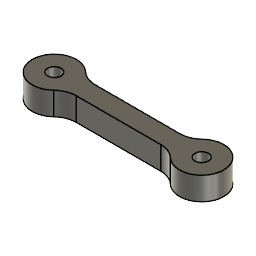
ConnectingBracketV0_v1 (Autodesk Fusion 360 design; units mm, degrees)
Autodesk Fusion 360 part; units mm, degrees
sketch "Sketch1" plane through (0, 0, 0) normal (0, 0, 1) x (1, 0, 0)
  line L0 (0, 0) -> (-19.119, 0) construction
  circle A0 centre (-19.119, 0) radius 0.875
  circle A1 centre (0, 0) radius 0.875
  line L1 (-9.5595, 0) -> (-9.5595, 1.25) construction
  line L2 (-9.5595, 0) -> (-9.5595, -1.25) construction
  line L3 (-19.119, 0) -> (-19.119, 0.875) construction
  line L4 (-19.119, 0.875) -> (-19.119, 2.875) construction
  circle A2 centre (-19.119, 0) radius 2.875
  line L5 (0, 0) -> (0, 0.875) construction
  line L6 (0, 0.875) -> (0, 2.875) construction
  circle A3 centre (0, 0) radius 2.875
  line L7 (-16.5237, 1.237) -> (-2.5953, 1.237)
  line L8 (-2.5953, 1.237) -> (-2.5953, -1.237) construction
  line L9 (-2.5953, -1.237) -> (-16.5237, -1.237)
  line L10 (-16.5237, -1.237) -> (-16.5237, 1.237) construction
  line L11 (-16.5237, 1.237) -> (-2.5953, -1.237) construction
  line L12 (-2.5953, 1.237) -> (-16.5237, -1.237) construction
  point P0 (-9.5595, 0)
  dimension "d9" = 19.119
  dimension "d10" = 1.75
  dimension "d11" = 1.75
  dimension "d12" = 1.25
  dimension "d13" = 1.25
  dimension "d14" = 2
  dimension "d15" = 2
  constraint coincident L0.start A1.centre
  constraint horizontal L0
  constraint coincident L0.end A0.centre
  constraint coincident L0 P0
  constraint perpendicular L0 L1
  constraint perpendicular L0 L2
  constraint coincident A0 L3.end
  constraint perpendicular L0 L3
  constraint perpendicular L0 L4
  constraint concentric A0 A2
  constraint coincident L4.end A2
  constraint coincident A1 L5.end
  constraint perpendicular L0 L5
  constraint vertical L6
  constraint coincident L6.end A3
  constraint horizontal L7
  constraint perpendicular L7 L8
  constraint parallel L7 L9
  constraint parallel L8 L10
  constraint coincident L11 P0
  constraint coincident L12 P0
  constraint coincident P0 L1.start
  constraint coincident A2 L7.start
  constraint coincident A3 L7.end
  measures "d9" distance of L0.start L0.end
  measures "d10" diameter of A0
  measures "d11" diameter of A1
  measures "d12" distance of P0 L1.end
  measures "d13" distance of P0 L2.end
  measures "d14" distance of L3.end L4.end
  measures "d15" distance of L5.end L6.end
extrude "Extrude2" add sketch "Sketch1" along normal blind 3
fillet "Fillet1" radius 3 4 edges at (-16.5237, -1.237, 1.5) (-2.5953, -1.237, 1.5) (-2.5953, 1.237, 1.5) (-16.5237, 1.237, 1.5)
equation "d12 = ( 2.5 / 2 ) * 1 mm"
